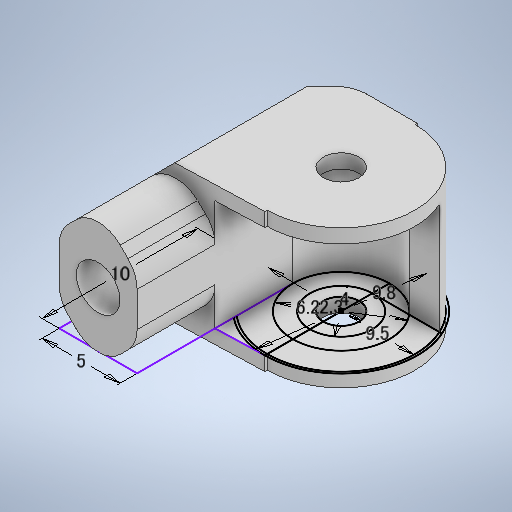
# Autodesk Inventor part: srod2.4_2.8
Saved by Autodesk Inventor 2025 (Build 290162000, 162)
## iProperties
Created: 2024-07-27
Part Number: srod2.4_2.8
Material: 一般
Document SubType Name: Modeling
Designer: Saigusa
Density: 1 g/cm^3
Appearance: 既定
Author: Saigusa
Autodesk Inventor part; units mm, degrees
ref_plane "YZ Plane" through (0, 0, 0) normal (1, 0, 0) x (0, 1, 0)
ref_plane "XZ Plane" through (0, 0, 0) normal (0, 1, 0) x (-1, 0, 0)
ref_plane "XY Plane" through (0, 0, 0) normal (0, 0, 1) x (1, 0, 0)
sketch "スケッチ1" plane through (0, 0, 0) normal (0, 1, 0) x (-1, 0, 0)
  circle A0 centre (0, 0) radius 1.15
  circle A1 centre (0, 0) radius 3.1
  circle A2 centre (0, 0) radius 4.9
  line L0 (3.1, 0) -> (8.1, 0)
  line L1 (8.1, 0) -> (8.1, 10)
  line L2 (8.1, 10) -> (3.1, 10)
  line L3 (3.1, 10) -> (3.1, 0)
  line L4 (0, 0) -> (0, 4.9)
  line L5 (0, 4.9) -> (3.1, 5)
  line L6 (8.1, 0) -> (2.9642, -3.9017)
  circle A3 centre (0, 0) radius 2
  line L7 (0, -2) -> (-4.4733, -2)
  line L8 (8.1, 0) -> (8.1, -4.9)
  line L9 (8.1, -4.9) -> (0, -4.9)
  circle A4 centre (0, 0) radius 4.75
  line L10 (0, 4.9) -> (0, -4.9)
  point P0 (-2.3685, -2)
  point P1 (-4.3084, -2)
  point P2 (0, -4.75)
  point P3 (0, 4.75)
  dimension "d1" = 6.2
  dimension "d5" = 4
  dimension "d0" = 2.3
  dimension "d2" = 9.8
  dimension "d3" = 5
  dimension "d4" = 10
  dimension "d29" = 9.5
  constraints: 22 end point, 5 coincident, 4 point on circle, 3 centre point, 2 horizontal, 2 parallel, 2 perpendicular, 2 tangent, 2 vertical, 1 collinear, 1 midpoint, 1 point on line, 1 vertical alignment, 5 other
  measures "d0" diameter of A0
  measures "d2" diameter of A2
  measures "d3" distance of L2.end L1.end
  measures "d4" distance of L1.end L0.end
  measures "d29" diameter of A4
extrude "押し出し1" add sketch "スケッチ1" along normal blind 7.1 contours A1 L10 A4 L7 | A1 L0 A4 L10 | L3 A4 L0 | A4 L0 A2 L10 | A4 L3 A2 L0 | A2 L6 L8 L9 | L0 L6 A2 | A2 L3 L2 L1 L0
extrude "押し出し2" add sketch "スケッチ1" against normal blind 0.9 contours A0 L4 A3 L10 | A0 L10 A3 L4 | A3 L7 A1 L4 | L4 A1 L10 A3 | L10 A1 L7 | L4 A4 L3 A1 | A1 L7 A4 L4 | A1 L10 A4 L7 | A1 L0 A4 L10 | L3 A4 L0 | L4 A2 L3 A4 | A4 L0 A2 L10 | A4 L3 A2 L0 | L5 L3 A2 | A2 L6 L8 L9 | L0 L6 A2 | A2 L3 L2 L1 L0
sketch "スケッチ2" plane through (0, 7.1, 0) normal (0, 1, 0) x (1, 0, 0)
  circle A0 centre (0, 0) radius 1.15 projected
  circle A1 centre (0, 0) radius 1.15
  arc A2 (2.3685, 2) -> (-3.1, 0) centre (0, 0) ccw projected
  circle A3 centre (0, 0) radius 4.9
  line L0 (-8.1, -10) -> (-8.1, 4.9) projected
  line L1 (-3.1, 0) -> (-8.1, 0)
  line L2 (-8.1, 0) -> (-8.1, -10)
  line L3 (-8.1, -10) -> (-3.1, -10)
  line L4 (-3.1, -10) -> (-3.1, 0)
  line L5 (-3.1, -5) -> (0, -4.9) projected
  line L6 (0, -4.9) -> (-3.1, -5)
  line L7 (-3.1, -5) -> (-3.1, 0)
  line L8 (0, 0) -> (-8.1, 0)
  line L9 (-8.1, 0) -> (-8.1, 4.9)
  line L10 (-8.1, 4.9) -> (0, 4.9)
  line L11 (0, 4.9) -> (0, 0)
  line L12 (0, -4.9) -> (0, 4.9)
  circle A4 centre (0, 0) radius 4.75
  point P0 (0, -4.75)
  point P1 (0, 4.75)
  dimension "d11" = 9.8
  dimension "d10" = 2.3
  dimension "d12" = 5
  dimension "d13" = 10
  dimension "d30" = 9.5
  constraints: 22 end point, 5 equal length, 3 coincident, 2 centre point, 2 horizontal, 2 perpendicular, 2 vertical, 1 tangent, 2 other
  measures "d10" diameter of A1
  measures "d12" distance of L3.end L0.start
  measures "d13" distance of L0.start L1.end
  measures "d30" diameter of A4
extrude "押し出し3" add sketch "スケッチ2" along normal blind 0.9 contours A0 L11 A4 L12 | A0 L8 A2 L11 | L12 A4 L4 L8 A0 | A2 L1 A4 L11 | L12 A3 L4 A4 | L4 A4 L1 | A4 L1 A3 L11 | L5 L4 A3 | L4 A3 L1 A4 | A3 L1 L0 L10 | L4 L3 L0 L1 A3
sketch "スケッチ3" plane through (-8.1, -0.9, 10) normal (0, 0, 1) x (1, 0, 0)
  line L0 (0, 0) -> (8.1, 0) projected
  line L1 (0, 0) -> (2.5, 0)
  line L2 (2.5, 0) -> (2.5, 4.425)
  line L3 (2.5, 4.425) -> (0, 4.425)
  line L4 (0, 4.425) -> (0, 0)
  circle A0 centre (2.5, 4.425) radius 1.6
  circle A1 centre (2.5, 4.425) radius 1.4
  point P0 (8.1, 0.9)
  point P1 (2.5, 3.025)
  point P2 (2.5, 2.825)
  point P3 (0.9, 4.425)
  point P4 (1.1, 4.425)
  dimension "d16" = 2.5
  dimension "d17" = 4.425
  dimension "d18" = 3.2
  dimension "d28" = 2.8
  constraints: 8 end point, 2 centre point, 2 coincident, 2 parallel, 1 horizontal, 1 perpendicular
  measures "d16" distance of L3.end L2.end
  measures "d17" distance of L2.end L1.end
  measures "d18" diameter of A0
  measures "d28" diameter of A1
extrude "押し出し4" cut sketch "スケッチ3" against normal blind 10 contours A1 L3 L2 | L2 L3 A1
chamfer "面取り1" distance 2.5 angle 45 4 edges at (-8.1, -0.9, 2.55) (-8.1, 8, 2.55) (-3.1, -0.9, 7.5) (-3.1, 8, 7.5)
chamfer "面取り3" distance 4 angle 45 1 edges at (-8.1, 3.55, -4.9)
fillet "フィレット2" radius 2 8 edges at (-4.1, 3.55, -4.9) (-8.1, 3.55, -0.9) (-5.6, 8, 7.5403) (-8.1, 5.5, 4.55) (-8.1, 1.6, 4.55) (-5.6, -0.9, 7.5403) (-3.1, 1.6, 7.5) (-3.1, 5.5, 7.5)
